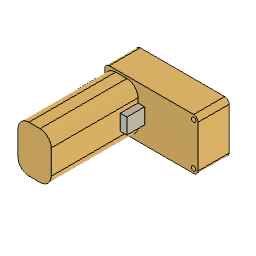
PeristalticPump_Gears (Autodesk Fusion 360 archive; units mm, degrees)
design "DC Motor from Hanka Dubovská"
part number: 2026-01-29-20-00-23-988
Autodesk Fusion 360 part; units mm, degrees
(part 1 of 2)
sketch "Sketch1" plane through (0, 0, 0) normal (0, 0, 1) x (1, 0, 0)
  line L0 (0, 0) -> (42, 0)
  line L1 (42, 0) -> (42, 14)
  line L2 (42, 14) -> (0, 14)
  line L3 (0, 14) -> (0, 0)
  line L4 (0, 0) -> (20, 0)
  dimension "d1" = 42
  dimension "d2" = 14
  constraint horizontal L0
  constraint vertical L1
  constraint horizontal L2
  constraint vertical L3
  constraint coincident L0.start L3.end
  constraint horizontal L4
  measures "d1" distance of L1.end L2.end
  measures "d2" distance of L0.end L1.end
extrude "Extrude1" add sketch "Sketch1" along normal blind 23
extrude "Extrude2" add sketch "Sketch1" along normal blind 22
sketch "Sketch3" plane through (0, 0, 0) normal (0, 1, 0) x (1, 0, 0)
  line L0 (15, -1) -> (0, -1)
  line L1 (0, -1) -> (0, -22)
  line L2 (0, -22) -> (15, -22)
  line L3 (15, -22) -> (15, -1)
  dimension "d17" = 15
  constraint horizontal L0
  constraint vertical L1
  constraint horizontal L2
  constraint vertical L3
  measures "d17" distance of L1.end L2.end
extrude "Extrude4" add sketch "Sketch3" against normal blind 39
fillet "Fillet2" radius 5 4 edges at (0, -19.5, 22) (15, -19.5, 22) (0, -19.5, 1) (15, -19.5, 1)
fillet "Fillet3" radius 2 4 edges at (0, 7, 0) (42, 7, 0) (42, 7, 23) (0, 7, 23)
sketch "Sketch4" plane through (0, 0, 0) normal (-1, 0, 0) x (0, -1, 0)
  line L0 (0, 21) -> (-14, 21)
  line L1 (-14, 21) -> (-14, 2)
  line L2 (-14, 2) -> (0, 2)
  line L3 (0, 2) -> (0, 6)
  line L4 (0, 6) -> (39, 6)
  line L5 (39, 6) -> (39, 17)
  line L6 (39, 17) -> (0, 17)
  line L7 (0, 17) -> (0, 21)
  line L8 (0, 15) -> (8, 15)
  line L9 (8, 15) -> (8, 8)
  line L10 (8, 8) -> (0, 8)
  line L11 (0, 8) -> (0, 15)
  dimension "d20" = 8
  dimension "d21" = 7
  constraint horizontal L8
  constraint vertical L9
  constraint horizontal L10
  constraint vertical L11
  measures "d20" distance of L8.start L8.end
  measures "d21" distance of L8.start L10.end
extrude "Extrude5" add sketch "Sketch4" along normal blind 4 contours L8 L9 L10 L11
sketch "Sketch5" plane through (0, 14, 0) normal (0, 1, 0) x (-1, 0, 0)
  arc A0 (0, 21) -> (-2, 23) centre (-2, 21) ccw
  line L0 (-2, 23) -> (-40, 23)
  arc A1 (-40, 23) -> (-42, 21) centre (-40, 21) ccw
  line L1 (-42, 21) -> (-42, 2)
  arc A2 (-42, 2) -> (-40, 0) centre (-40, 2) ccw
  line L2 (-40, 0) -> (-2, 0)
  arc A3 (-2, 0) -> (0, 2) centre (-2, 2) ccw
  line L3 (0, 2) -> (0, 21)
  line L4 (-30.8362, 13.6553) -> (-29.8362, 13.6553)
  line L5 (-28.8362, 12.6553) -> (-28.8362, 9.6553)
  line L6 (-29.8362, 8.6553) -> (-30.8362, 8.6553)
  line L7 (-31.8362, 9.6553) -> (-31.8362, 12.6553)
  circle A4 centre (-21, 11.5403) radius 1.5
  arc A5 (-28.8362, 12.6553) -> (-29.8362, 13.6553) centre (-29.8362, 12.6553) ccw
  arc A6 (-30.8362, 13.6553) -> (-31.8362, 12.6553) centre (-30.8362, 12.6553) ccw
  arc A7 (-31.8362, 9.6553) -> (-30.8362, 8.6553) centre (-30.8362, 9.6553) ccw
  arc A8 (-29.8362, 8.6553) -> (-28.8362, 9.6553) centre (-29.8362, 9.6553) ccw
  point P0 (-28.8362, 13.6553)
  point P1 (-28.8362, 8.6553)
  point P2 (-31.8362, 8.6553)
  dimension "d24" = 3
  dimension "d25" = 5
  dimension "d26" = 3
  dimension "d37" = 1
  constraint horizontal L4
  constraint vertical L5
  constraint horizontal L6
  constraint vertical L7
  constraint coincident P0 L4
  constraint coincident P0 L5
  constraint tangent L4 A5
  constraint tangent L5 A5
  constraint tangent L4 A6
  constraint tangent L7 A6
  constraint equal A5 A6
  constraint coincident P2 L6
  constraint coincident P2 L7
  constraint tangent L6 A7
  constraint tangent L7 A7
  constraint equal A5 A7
  constraint coincident P1 L5
  constraint coincident P1 L6
  constraint tangent L5 A8
  constraint tangent L6 A8
  constraint equal A5 A8
  measures "d24" diameter of A4
  measures "d25" distance of P0 P1
  measures "d26" distance of P1 P2
  measures "d37" radius of A5
extrude "Extrude6" add sketch "Sketch5" along normal blind 8 contours L4 L5 L6 L7 A5 A6 A7 A8
sketch "Sketch6" plane through (0, 14, 0) normal (0, 1, 0) x (-1, 0, 0)
  circle A0 centre (-21, 11.5) radius 1.5
  dimension "d29" = 3
  measures "d29" diameter of A0
extrude "Extrude7" add sketch "Sketch6" along normal blind 1
sketch "Sketch7" plane through (15, 0, 0) normal (1, 0, 0) x (0, 1, 0)
  line L0 (-39, 6) -> (0, 6)
  line L1 (0, 6) -> (0, 17)
  line L2 (0, 17) -> (-39, 17)
  line L3 (-39, 17) -> (-39, 6)
  line L4 (0, 15) -> (-8, 15)
  line L5 (-8, 15) -> (-8, 8)
  line L6 (-8, 8) -> (0, 8)
  line L7 (0, 8) -> (0, 15)
  constraint horizontal L4
  constraint vertical L5
  constraint horizontal L6
  constraint vertical L7
  constraint coincident L1 L4.start
extrude "Extrude8" add sketch "Sketch7" along normal blind 3 contours L1 L4 L5 L6 L7
sketch "Sketch8" plane through (0, 14, 0) normal (0, 1, 0) x (-1, 0, 0)
  circle A0 centre (-21, 11.5) radius 1.5
  line L0 (-31.8362, 9.6553) -> (-31.8362, 12.6553)
  line L1 (-30.8362, 13.6553) -> (-29.8362, 13.6553)
  line L2 (-28.8362, 12.6553) -> (-28.8362, 9.6553)
  line L3 (-29.8362, 8.6553) -> (-30.8362, 8.6553)
  arc A1 (0, 21) -> (-2, 23) centre (-2, 21) ccw
  line L4 (-2, 23) -> (-40, 23)
  arc A2 (-40, 23) -> (-42, 21) centre (-40, 21) ccw
  line L5 (-42, 21) -> (-42, 2)
  arc A3 (-42, 2) -> (-40, 0) centre (-40, 2) ccw
  line L6 (-40, 0) -> (-2, 0)
  arc A4 (-2, 0) -> (0, 2) centre (-2, 2) ccw
  line L7 (0, 2) -> (0, 21)
  circle A5 centre (-40, 2) radius 1
  circle A6 centre (-40, 21) radius 1
  arc A7 (-30.8362, 13.6553) -> (-31.8362, 12.6553) centre (-30.8362, 12.6553) ccw
  arc A8 (-28.8362, 12.6553) -> (-29.8362, 13.6553) centre (-29.8362, 12.6553) ccw
  arc A9 (-29.8362, 8.6553) -> (-28.8362, 9.6553) centre (-29.8362, 9.6553) ccw
  arc A10 (-31.8362, 9.6553) -> (-30.8362, 8.6553) centre (-30.8362, 9.6553) ccw
  constraint concentric A3 A5
  constraint concentric A2 A6
hole "Hole1" at (40, 14, 2) at (40, 14, 21) direction (0, -1, 0) diameter 2 depth 14 tip angle 118

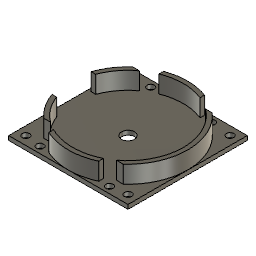
design "GearHolder"
part number: 2026-05-20-10-56-44-048
Autodesk Fusion 360 part; units mm, degrees
sketch "Sketch1" plane through (0, 0, 0) normal (0, 0, 1) x (1, 0, 0)
  line L0 (0, 55) -> (0, 0)
  circle A0 centre (51, 51) radius 1.65
  circle A1 centre (4, 51) radius 1.65
  line L1 (25, 0) -> (30, 0)
  line L2 (0, 0) -> (55, 0)
  line L3 (55, 55) -> (0, 55)
  circle A2 centre (4, 4) radius 1.65
  circle A3 centre (51, 4) radius 1.65
  line L4 (55, 0) -> (55, 55)
  line L5 (45, 55) -> (9.9854, 55)
  line L6 (45, 55) -> (38, 55)
  circle A4 centre (11.5, 3) radius 1.65
  line L7 (16.9854, 55) -> (9.9854, 55)
  circle A5 centre (43.5, 3) radius 1.65
  line L8 (8, 0) -> (47, 0)
  circle A6 centre (13.4854, 52) radius 1.65
  circle A7 centre (41.5, 52) radius 1.65
  circle A8 centre (27.5, 27.5) radius 3
  point P0 (45, 45)
  dimension "d30" = 3.3
  dimension "d31" = 4
  dimension "d32" = 4
  dimension "d33" = 3.3
  dimension "d34" = 4
  dimension "d35" = 4
  dimension "d36" = 3.3
  dimension "d37" = 4
  dimension "d38" = 4
  dimension "d39" = 3.3
  dimension "d40" = 4
  dimension "d41" = 4
  dimension "d55" = 3.3
  dimension "d56" = 3.3
  dimension "d57" = 3
  dimension "d59" = 3
  dimension "d60" = 3.3
  dimension "d61" = 3.3
  dimension "d62" = 3
  dimension "d65" = 3
  dimension "d69" = 6
  dimension "d70" = 55
  dimension "d71" = 27.5
  dimension "d72" = 55
  dimension "d73" = 27.5
  constraint horizontal L2
  constraint vertical L4
  constraint horizontal L3
  constraint vertical L0
  constraint horizontal L1
  constraint coincident L1.start L2
  constraint coincident L5.start L6.start
  constraint coincident L5.end L7.end
  measures "d30" diameter of A2
  measures "d31" distance of A2.centre L2
  measures "d32" distance of A2.centre L0
  measures "d33" diameter of A3
  measures "d34" distance of A3.centre L2
  measures "d35" distance of A3.centre L4
  measures "d36" diameter of A1
  measures "d37" distance of A1.centre L3
  measures "d38" distance of A1.centre L0
  measures "d39" diameter of A0
  measures "d40" distance of A0.centre L3
  measures "d41" distance of A0.centre L4
  measures "d55" diameter of A7
  measures "d56" diameter of A6
  measures "d57" distance of A7.centre L5
  measures "d59" distance of A6.centre L5
  measures "d60" diameter of A5
  measures "d61" diameter of A4
  measures "d62" distance of A5.centre L8
  measures "d65" distance of A4.centre L8
  measures "d69" diameter of A8
  measures "d70" distance of L0.start L0.end
  measures "d71" distance of L3 A8.centre
  measures "d72" distance of L0.start L3.start
  measures "d73" distance of L4 A8.centre
extrude "Extrude1" add sketch "Sketch1" along normal blind 2
sketch "Sketch2" plane through (0, 0, 2) normal (0, 0, 1) x (-1, 0, 0)
  line L0 (0, 0) -> (-55, 0)
  line L1 (-55, 0) -> (-55, -55)
  line L2 (-55, -55) -> (0, -55)
  line L3 (0, -55) -> (0, 0)
  circle A0 centre (-51, -51) radius 1.65
  circle A1 centre (-4, -51) radius 1.65
  circle A2 centre (-51, -4) radius 1.65
  circle A3 centre (-13.4854, -52) radius 1.65
  circle A4 centre (-43.5, -3) radius 1.65
  circle A5 centre (-4, -4) radius 1.65
  circle A6 centre (-41.5, -52) radius 1.65
  circle A7 centre (-11.5, -3) radius 1.65
  circle A8 centre (-27.5, -27.5) radius 3
  circle A9 centre (-27.5, -27.5) radius 27.5
  circle A10 centre (-27.5, -27.5) radius 25.5
  line L4 (-18, -48) -> (-8.9708, -48)
  line L5 (-8.9708, -48) -> (-8.9708, -56)
  line L6 (-8.9708, -56) -> (-18, -56)
  line L7 (-18, -56) -> (-18, -48)
  line L8 (-18, -48) -> (-8.9708, -56) construction
  line L9 (-8.9708, -48) -> (-18, -56) construction
  line L10 (-37, -48) -> (-46, -48)
  line L11 (-46, -48) -> (-46, -56)
  line L12 (-46, -56) -> (-37, -56)
  line L13 (-37, -56) -> (-37, -48)
  line L14 (-37, -48) -> (-46, -56) construction
  line L15 (-46, -48) -> (-37, -56) construction
  line L16 (-39, -7) -> (-48, -7)
  line L17 (-48, -7) -> (-48, 1)
  line L18 (-48, 1) -> (-39, 1)
  line L19 (-39, 1) -> (-39, -7)
  line L20 (-39, -7) -> (-48, 1) construction
  line L21 (-48, -7) -> (-39, 1) construction
  line L22 (-16, -7) -> (-7, -7)
  line L23 (-7, -7) -> (-7, 1)
  line L24 (-7, 1) -> (-16, 1)
  line L25 (-16, 1) -> (-16, -7)
  line L26 (-16, -7) -> (-7, 1) construction
  line L27 (-7, -7) -> (-16, 1) construction
  line L28 (0, -36.5) -> (-10, -36.5)
  line L29 (-10, -36.5) -> (-10, -18.5)
  line L30 (-10, -18.5) -> (0, -18.5)
  line L31 (0, -18.5) -> (0, -36.5)
  point P0 (-13.4854, -52)
  point P1 (-41.5, -52)
  point P2 (-43.5, -3)
  point P3 (-11.5, -3)
  dimension "d74" = 2
  dimension "d75" = 51
  dimension "d78" = 18
  dimension "d79" = 18.5
  constraint concentric A8 A9
  constraint concentric A8 A10
  constraint horizontal L4
  constraint perpendicular L4 L5
  constraint parallel L4 L6
  constraint parallel L5 L7
  constraint coincident L8 P0
  constraint coincident L9 P0
  constraint coincident P0 A3.centre
  constraint horizontal L10
  constraint perpendicular L10 L11
  constraint parallel L10 L12
  constraint parallel L11 L13
  constraint coincident L14 P1
  constraint coincident L15 P1
  constraint coincident P1 A6.centre
  constraint horizontal L16
  constraint perpendicular L16 L17
  constraint parallel L16 L18
  constraint parallel L17 L19
  constraint coincident L20 P2
  constraint coincident L21 P2
  constraint coincident P2 A4.centre
  constraint horizontal L22
  constraint perpendicular L22 L23
  constraint parallel L22 L24
  constraint parallel L23 L25
  constraint coincident L26 P3
  constraint coincident L27 P3
  constraint coincident P3 A7.centre
  constraint horizontal L28
  constraint vertical L29
  constraint horizontal L30
  constraint vertical L31
  constraint coincident L3 L28.start
  measures "d74" distance of A9 A10
  measures "d75" diameter of A10
  measures "d78" distance of L28.end L29.end
  measures "d79" distance of L2.end L28.start
extrude "Extrude2" add sketch "Sketch2" along normal blind 8 contours A9 A10 L22 L30 | A9 A10 L19 L25 | A9 A10 L4 L28 | A9 A10 L10 L16 | A9 A10 L7 L13

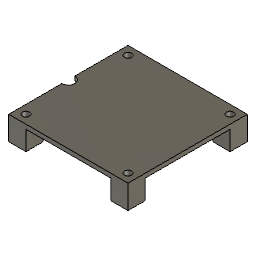
design "GearHolderP2"
part number: 2026-05-20-11-23-21-013
Autodesk Fusion 360 part; units mm, degrees
sketch "Sketch1" plane through (0, 0, 0) normal (0, 0, 1) x (1, 0, 0)
  circle A0 centre (51, 4) radius 1.65
  line L0 (16.9854, 55) -> (9.9854, 55)
  line L1 (0, 55) -> (0, 0)
  circle A1 centre (4, 4) radius 1.65
  line L2 (25, 0) -> (30, 0)
  line L3 (8, 0) -> (47, 0)
  line L4 (55, 0) -> (55, 55)
  line L5 (0, 0) -> (55, 0)
  line L6 (45, 55) -> (38, 55)
  line L7 (55, 55) -> (0, 55)
  circle A2 centre (51, 51) radius 1.65
  circle A3 centre (4, 51) radius 1.65
  line L8 (45, 55) -> (9.9854, 55)
  line L9 (0, 55) -> (8, 55)
  line L10 (8, 55) -> (8, 47)
  line L11 (8, 47) -> (0, 47)
  line L12 (0, 47) -> (0, 55)
  line L13 (0, 55) -> (8, 47) construction
  line L14 (8, 55) -> (0, 47) construction
  line L15 (55, 55) -> (47, 55)
  line L16 (47, 55) -> (47, 47)
  line L17 (47, 47) -> (55, 47)
  line L18 (55, 47) -> (55, 55)
  line L19 (55, 55) -> (47, 47) construction
  line L20 (47, 55) -> (55, 47) construction
  line L21 (55, 0) -> (47, 0)
  line L22 (47, 0) -> (47, 8)
  line L23 (47, 8) -> (55, 8)
  line L24 (55, 8) -> (55, 0)
  line L25 (55, 0) -> (47, 8) construction
  line L26 (47, 0) -> (55, 8) construction
  line L27 (0, 0) -> (8, 0)
  line L28 (8, 0) -> (8, 8)
  line L29 (8, 8) -> (0, 8)
  line L30 (0, 8) -> (0, 0)
  line L31 (0, 0) -> (8, 8) construction
  line L32 (8, 0) -> (0, 8) construction
  circle A4 centre (0, 27.5) radius 3
  point P0 (45, 45)
  point P1 (4, 51)
  point P2 (51, 51)
  point P3 (51, 4)
  point P4 (4, 4)
  dimension "d1" = 3.3
  dimension "d2" = 4
  dimension "d3" = 4
  dimension "d4" = 3.3
  dimension "d5" = 4
  dimension "d6" = 4
  dimension "d7" = 3.3
  dimension "d8" = 4
  dimension "d9" = 4
  dimension "d10" = 3.3
  dimension "d11" = 4
  dimension "d12" = 4
  dimension "d22" = 55
  dimension "d24" = 55
  dimension "d31" = 6
  dimension "d32" = 27.5
  constraint horizontal L5
  constraint vertical L4
  constraint horizontal L7
  constraint vertical L1
  constraint horizontal L2
  constraint coincident L2.start L5
  constraint coincident L6.start L8.start
  constraint coincident L0.end L8.end
  constraint horizontal L9
  constraint perpendicular L9 L10
  constraint parallel L9 L11
  constraint parallel L10 L12
  constraint coincident L13 P1
  constraint coincident L14 P1
  constraint coincident P1 A3.centre
  constraint horizontal L15
  constraint perpendicular L15 L16
  constraint parallel L15 L17
  constraint parallel L16 L18
  constraint coincident L19 P2
  constraint coincident L20 P2
  constraint coincident P2 A2.centre
  constraint horizontal L21
  constraint perpendicular L21 L22
  constraint parallel L21 L23
  constraint parallel L22 L24
  constraint coincident L25 P3
  constraint coincident L26 P3
  constraint coincident A0.centre P3
  constraint horizontal L27
  constraint perpendicular L27 L28
  constraint parallel L27 L29
  constraint parallel L28 L30
  constraint coincident L31 P4
  constraint coincident L32 P4
  constraint coincident L1.end L5.start
  constraint coincident P4 A1.centre
  constraint coincident L1 A4.centre
  measures "d1" diameter of A1
  measures "d2" distance of P4 L5
  measures "d3" distance of P4 L1
  measures "d4" diameter of A0
  measures "d5" distance of A0.centre L5
  measures "d6" distance of A0.centre L4
  measures "d7" diameter of A3
  measures "d8" distance of P1 L7
  measures "d9" distance of P1 L1
  measures "d10" diameter of A2
  measures "d11" distance of P2 L7
  measures "d12" distance of P2 L4
  measures "d22" distance of L1.start L1.end
  measures "d24" distance of L1.start L4.end
  measures "d31" diameter of A4
  measures "d32" distance of L1.start A4.centre
extrude "Extrude1" add sketch "Sketch1" along normal blind 9 contours L1 L7 L9 L10 L11 L12 | L4 L7 L15 L16 L17 L18 | L4 L5 L21 L22 L23 L24 | L1 L5 L27 L28 L29 L30 makes body 1 at (50.1048, 49.614, 6) makes body 2 at (51.8952, 2.614, 3) makes body 3 at (5.6173, 50.6731, 6) makes body 4 at (5.6479, 3.9178, 6)
extrude "Extrude2" add sketch "Sketch1" along normal blind 2 from surface at 9 contours L0 L1 L2 L3 L4 L5 L6 L7 L8 L10 L11 L16 L17 L22 L23 L28 L29 A4 | L1 L7 L9 L10 L11 L12 | L4 L7 L15 L16 L17 L18 | L4 L5 L21 L22 L23 L24 | L1 L5 L27 L28 L29 L30 bodies 1 2 3 4

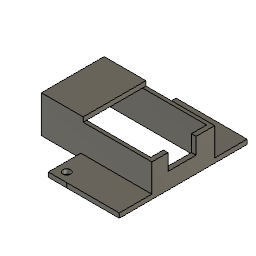
design "GearHolderP3"
part number: 2026-05-20-11-42-52-176
Autodesk Fusion 360 part; units mm, degrees
sketch "Sketch1" plane through (0, 0, 0) normal (0, 0, 1) x (1, 0, 0)
  line L0 (0, 55) -> (-8, 47) construction
  circle A0 centre (-4.0079, 4.0002) radius 1.65
  line L1 (-0.0158, 8.0004) -> (-8, 8.0004)
  line L2 (-8, 0) -> (-0.0158, 8.0004) construction
  line L3 (-0.0158, 0) -> (-8, 8.0004) construction
  line L4 (-0.0158, 0) -> (-0.0158, 8.0004)
  line L5 (0, 55) -> (0, 47)
  line L6 (-8, 0) -> (-0.0158, 0)
  line L7 (-8, 8.0004) -> (-8, 0)
  line L8 (-8, 47) -> (-8, 55)
  circle A1 centre (-4, 51) radius 1.65
  line L9 (-8, 55) -> (0, 47) construction
  line L10 (-8, 55) -> (0, 55)
  line L11 (0, 47) -> (-8, 47)
  line L12 (20.5318, 39.5004) -> (20.5318, 15.5004)
  line L13 (20.5318, 39.5004) -> (-23, 39.5004)
  line L14 (-22.9682, 39.5004) -> (-22.9682, 15.5004)
  line L15 (-22.9682, 15.5004) -> (20.5318, 15.5004)
  line L16 (-24.9682, 41.0004) -> (22.5318, 41.0004)
  line L17 (22.5318, 41.0004) -> (22.5318, 14.0004)
  line L18 (22.5318, 14.0004) -> (-24.9682, 14.0004)
  line L19 (-24.9682, 14.0004) -> (-24.9682, 41.0004)
  line L20 (-6.9682, 41.0004) -> (-6.9682, 14.0004)
  line L21 (-8, 47) -> (-8, 41)
  line L22 (-8, 8.0004) -> (-8, 14.0004)
  line L23 (22.5318, 41.0004) -> (22.5318, 54.9634)
  line L24 (22.5318, 54.9634) -> (0, 55)
  line L25 (22.5318, 14.0004) -> (22.5318, -0.0052)
  line L26 (22.5318, -0.0052) -> (-0.0158, 0)
  line L27 (20.5318, 33) -> (22.5318, 33)
  line L28 (22.5318, 33) -> (22.5318, 21)
  line L29 (22.5318, 21) -> (20.5318, 21)
  line L30 (20.5318, 21) -> (20.5318, 33)
  point P0 (-8, 0)
  point P1 (-4, 51)
  point P2 (-4.0079, 4.0002)
  point P3 (9.9854, 55)
  point P4 (9.9854, 55)
  point P5 (-7.9947, 0.536)
  point P6 (-0.0158, 0)
  dimension "d1" = 3.3
  dimension "d3" = 3.3
  dimension "d6" = 24
  dimension "d8" = 1.5
  dimension "d9" = 2
  dimension "d10" = 1.5
  dimension "d11" = 2
  dimension "d12" = 16
  dimension "d14" = 8
  dimension "d15" = 8
  dimension "d18" = 6
  dimension "d19" = 6
  dimension "d20" = 8.0004
  dimension "d30" = 43.5
  constraint coincident P4 P3
  constraint horizontal L10
  constraint perpendicular L5 L10
  constraint parallel L10 L11
  constraint parallel L5 L8
  constraint coincident P1 L9
  constraint coincident P1 L0
  constraint coincident P1 A1.centre
  constraint horizontal L6
  constraint perpendicular L4 L6
  constraint parallel L1 L6
  constraint parallel L4 L7
  constraint coincident P2 L2
  constraint coincident P2 L3
  constraint coincident P0 L2.start
  constraint coincident P2 A0.centre
  constraint perpendicular L12 L13
  constraint coincident L13 L14.start
  constraint perpendicular L13 L14
  constraint horizontal L16
  constraint vertical L17
  constraint horizontal L18
  constraint vertical L19
  constraint coincident L16 L20.start
  constraint coincident L18 L20.end
  constraint perpendicular L18 L20
  constraint perpendicular L16 L21
  constraint coincident L18 L22.end
  constraint perpendicular L18 L22
  constraint perpendicular L16 L23
  constraint perpendicular L18 L25
  constraint coincident P6 L3.start
  constraint horizontal L27
  constraint vertical L28
  constraint horizontal L29
  constraint vertical L30
  constraint coincident L17 L28.end
  constraint coincident L12 L27.start
  measures "d1" diameter of A0
  measures "d3" diameter of A1
  measures "d6" distance of L12.start L12.end
  measures "d8" distance of L13 L16
  measures "d9" distance of L12 L17
  measures "d10" distance of L15 L18
  measures "d11" distance of L14 L19
  measures "d12" distance of L14 L20
  measures "d14" distance of L8.end L0.start
  measures "d15" distance of L8.end L0.end
  measures "d18" distance of L0.end L21.end
  measures "d19" distance of L1.end L22.end
  measures "d20" distance of L1.end P0
  measures "d30" distance of L12 L14
extrude "Extrude1" add sketch "Sketch1" along normal blind 2 contours L1 L4 L6 L7 | L1 L4 L18 L22 L25 L26 | L5 L11 L16 L21 L23 L24 | L5 L8 L10 L11 makes body 1 at (15.0212, 50.3213, 0) makes body 2 at (15.0159, 4.6651, 0)
extrude "Extrude2" add sketch "Sketch1" along normal blind 14 contours L13 L14 L15 L16 L18 L19 L20 | L12 L15 L17 L18 L20 L29 | L12 L13 L16 L17 L20 L27 bodies 1 2
extrude "Extrude3" add sketch "Sketch1" along normal blind 2 from surface at 14 contours L13 L14 L15 L16 L18 L19 L20 | L13 L14 L15 L20 bodies 1
extrude "Extrude4" add sketch "Sketch1" along normal blind 7 contours L12 L17 L27 L28 L29 L30 bodies 1

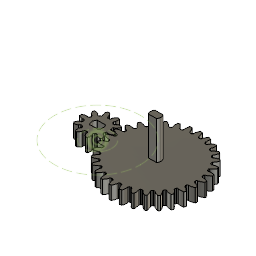
design "MotorGearsV3"
description: Spur Gear; Module: 1.5; Num Teeth: 30; Pressure Angle: 20.0; Backlash: 0.00 mm
part number: 2026-05-20-09-17-09-807
Autodesk Fusion 360 part; units mm, degrees
sketch "Base Circle" plane through (0, 0, 0) normal (0, 0, 1) x (1, 0, 0)
  circle A0 centre (0, 0) radius 5.7645
extrude "Extrude1" add sketch "Base Circle" along normal blind 7 makes body 1
sketch "Gear Tooth" plane through (0, 0, 0) normal (0, 0, 1) x (1, 0, 0)
  spline S0 degree 5 poles (6.9437, -1.2061) (6.9494, -1.2071) (6.9609, -1.2089) (6.9781, -1.211) (7.0011, -1.2127) (7.0301, -1.2132) (7.0593, -1.2127) (7.0885, -1.2115) (7.1178, -1.2099) (7.1471, -1.208) (7.1764, -1.2059) (7.2058, -1.2034) (7.2353, -1.2005) (7.2647, -1.197) (7.2943, -1.1929) (7.3238, -1.1884) (7.3534, -1.1833) (7.383, -1.178) (7.4126, -1.1723) (7.4422, -1.1663) (7.4719, -1.1599) (7.5015, -1.1533) (7.5312, -1.1463) (7.5609, -1.139) (7.5906, -1.1313) (7.6202, -1.1232) (7.6499, -1.1148) (7.6796, -1.1062) (7.7093, -1.0972) (7.7389, -1.0879) (7.7686, -1.0784) (7.7983, -1.0685) (7.8279, -1.0584) (7.8575, -1.048) (7.8872, -1.0372) (7.9168, -1.0262) (7.9464, -1.015) (7.9759, -1.0034) (8.0055, -0.9916) (8.035, -0.9795) (8.0645, -0.9671) (8.094, -0.9545) (8.1235, -0.9416) (8.1529, -0.9284) (8.1823, -0.915) (8.2117, -0.9013) (8.241, -0.8874) (8.2704, -0.8732) (8.2996, -0.8587) (8.3289, -0.844) (8.3581, -0.8291) (8.3873, -0.8139) (8.4164, -0.7985) (8.4455, -0.7828) (8.4746, -0.7669) (8.5036, -0.7508) (8.5325, -0.7344) (8.5615, -0.7177) (8.5903, -0.7009) (8.6192, -0.6838) (8.648, -0.6664) (8.6767, -0.6489) (8.7054, -0.6311) (8.734, -0.613) (8.7626, -0.5948) (8.7911, -0.5763) (8.8196, -0.5576) (8.848, -0.5387) (8.8764, -0.5195) (8.9047, -0.5001) (8.9329, -0.4805) (8.9555, -0.4647) (8.9723, -0.4527) (8.9836, -0.4446) (8.9892, -0.4406) knots 0 0 0 0 0 0 0.01428571 0.02857143 0.04285714 0.05714286 0.07142857 0.08571429 0.1 0.11428571 0.12857143 0.14285714 0.15714286 0.17142857 0.18571429 0.2 0.21428571 0.22857143 0.24285714 0.25714286 0.27142857 0.28571429 0.3 0.31428571 0.32857143 0.34285714 0.35714286 0.37142857 0.38571429 0.4 0.41428571 0.42857143 0.44285714 0.45714286 0.47142857 0.48571429 0.5 0.51428571 0.52857143 0.54285714 0.55714286 0.57142857 0.58571429 0.6 0.61428571 0.62857143 0.64285714 0.65714286 0.67142857 0.68571429 0.7 0.71428571 0.72857143 0.74285714 0.75714286 0.77142857 0.78571429 0.8 0.81428571 0.82857143 0.84285714 0.85714286 0.87142857 0.88571429 0.9 0.91428571 0.92857143 0.94285714 0.95714286 0.97142857 0.98571429 1 1 1 1 1 1
  spline S1 degree 5 poles (6.9437, 1.2061) (6.9494, 1.2071) (6.9609, 1.2089) (6.9781, 1.211) (7.0011, 1.2127) (7.0301, 1.2132) (7.0593, 1.2127) (7.0885, 1.2115) (7.1178, 1.2099) (7.1471, 1.208) (7.1764, 1.2059) (7.2058, 1.2034) (7.2353, 1.2005) (7.2647, 1.197) (7.2943, 1.1929) (7.3238, 1.1884) (7.3534, 1.1833) (7.383, 1.178) (7.4126, 1.1723) (7.4422, 1.1663) (7.4719, 1.1599) (7.5015, 1.1533) (7.5312, 1.1463) (7.5609, 1.139) (7.5906, 1.1313) (7.6202, 1.1232) (7.6499, 1.1148) (7.6796, 1.1062) (7.7093, 1.0972) (7.7389, 1.0879) (7.7686, 1.0784) (7.7983, 1.0685) (7.8279, 1.0584) (7.8575, 1.048) (7.8872, 1.0372) (7.9168, 1.0262) (7.9464, 1.015) (7.9759, 1.0034) (8.0055, 0.9916) (8.035, 0.9795) (8.0645, 0.9671) (8.094, 0.9545) (8.1235, 0.9416) (8.1529, 0.9284) (8.1823, 0.915) (8.2117, 0.9013) (8.241, 0.8874) (8.2704, 0.8732) (8.2996, 0.8587) (8.3289, 0.844) (8.3581, 0.8291) (8.3873, 0.8139) (8.4164, 0.7985) (8.4455, 0.7828) (8.4746, 0.7669) (8.5036, 0.7508) (8.5325, 0.7344) (8.5615, 0.7177) (8.5903, 0.7009) (8.6192, 0.6838) (8.648, 0.6664) (8.6767, 0.6489) (8.7054, 0.6311) (8.734, 0.613) (8.7626, 0.5948) (8.7911, 0.5763) (8.8196, 0.5576) (8.848, 0.5387) (8.8764, 0.5195) (8.9047, 0.5001) (8.9329, 0.4805) (8.9555, 0.4647) (8.9723, 0.4527) (8.9836, 0.4446) (8.9892, 0.4406) knots 0 0 0 0 0 0 0.01428571 0.02857143 0.04285714 0.05714286 0.07142857 0.08571429 0.1 0.11428571 0.12857143 0.14285714 0.15714286 0.17142857 0.18571429 0.2 0.21428571 0.22857143 0.24285714 0.25714286 0.27142857 0.28571429 0.3 0.31428571 0.32857143 0.34285714 0.35714286 0.37142857 0.38571429 0.4 0.41428571 0.42857143 0.44285714 0.45714286 0.47142857 0.48571429 0.5 0.51428571 0.52857143 0.54285714 0.55714286 0.57142857 0.58571429 0.6 0.61428571 0.62857143 0.64285714 0.65714286 0.67142857 0.68571429 0.7 0.71428571 0.72857143 0.74285714 0.75714286 0.77142857 0.78571429 0.8 0.81428571 0.82857143 0.84285714 0.85714286 0.87142857 0.88571429 0.9 0.91428571 0.92857143 0.94285714 0.95714286 0.97142857 0.98571429 1 1 1 1 1 1
  arc A0 (8.9892, -0.4406) -> (8.9892, 0.4406) centre (0, 0) ccw
  line L0 (5.6696, -0.9848) -> (6.9437, -1.2061)
  line L1 (5.6696, 0.9848) -> (6.9437, 1.2061)
  line L2 (5.6696, -0.9848) -> (5.6696, 0.9848)
  point P0 (7.0843, -1.2116)
  point P1 (7.2275, -1.2012)
  point P2 (7.3722, -1.1799)
  point P3 (7.5182, -1.1493)
  point P4 (7.6649, -1.1104)
  point P5 (7.8123, -1.0637)
  point P6 (7.9601, -1.0096)
  point P7 (8.108, -0.9483)
  point P8 (8.256, -0.8801)
  point P9 (8.4037, -0.8052)
  point P10 (8.5511, -0.7237)
  point P11 (8.6979, -0.6357)
  point P12 (8.844, -0.5413)
  point P13 (7.0843, 1.2116)
  point P14 (7.2275, 1.2012)
  point P15 (7.3722, 1.1799)
  point P16 (7.5182, 1.1493)
  point P17 (7.6649, 1.1104)
  point P18 (7.8123, 1.0637)
  point P19 (7.9601, 1.0096)
  point P20 (8.108, 0.9483)
  point P21 (8.256, 0.8801)
  point P22 (8.4037, 0.8052)
  point P23 (8.5511, 0.7237)
  point P24 (8.6979, 0.6357)
  point P25 (8.844, 0.5413)
extrude "Extrude2" add sketch "Gear Tooth" along normal blind 7 bodies 1
fillet "Fillet1" radius 0.5 2 edges at (5.6795, -0.9865, 3.5) (5.6795, 0.9865, 3.5) on bodies 1
pattern_circular "C-Pattern1" count 10 over 360 about axis through (0, 0, 0) along (0, 0, 1) of "Extrude2", "Fillet1"
sketch "Diametrial Pitch Circle" plane through (0, 0, 0) normal (0, 0, 1) x (1, 0, 0)
  circle A0 centre (0, 0) radius 7.5 construction
sketch "Base Circle (1)" plane through (0, 0, 0) normal (0, 0, 1) x (1, 0, 0)
  circle A0 centre (0, 0) radius 20.7645
extrude "Extrude3" add sketch "Base Circle (1)" along normal blind 7 separate body makes body 2
sketch "Gear Tooth (1)" plane through (0, 0, 0) normal (0, 0, 1) x (1, 0, 0)
  spline S0 degree 5 poles (21.0953, -1.4211) (21.1036, -1.4217) (21.1202, -1.4226) (21.1452, -1.4234) (21.1786, -1.4233) (21.2203, -1.4217) (21.262, -1.419) (21.3037, -1.4156) (21.3455, -1.4119) (21.3873, -1.4079) (21.4291, -1.4036) (21.4709, -1.399) (21.5127, -1.3939) (21.5545, -1.3883) (21.5963, -1.3822) (21.6381, -1.3756) (21.6799, -1.3685) (21.7217, -1.3611) (21.7635, -1.3534) (21.8052, -1.3454) (21.847, -1.3371) (21.8888, -1.3285) (21.9306, -1.3196) (21.9723, -1.3103) (22.014, -1.3008) (22.0558, -1.2909) (22.0975, -1.2807) (22.1392, -1.2702) (22.1809, -1.2594) (22.2225, -1.2484) (22.2642, -1.2371) (22.3059, -1.2255) (22.3475, -1.2137) (22.3891, -1.2016) (22.4307, -1.1893) (22.4723, -1.1767) (22.5138, -1.1638) (22.5554, -1.1507) (22.5969, -1.1374) (22.6384, -1.1238) (22.6799, -1.11) (22.7213, -1.0959) (22.7628, -1.0816) (22.8042, -1.0671) (22.8456, -1.0523) (22.887, -1.0373) (22.9283, -1.0221) (22.9696, -1.0067) (23.0109, -0.991) (23.0522, -0.9751) (23.0934, -0.959) (23.1347, -0.9427) (23.1759, -0.9262) (23.217, -0.9095) (23.2582, -0.8925) (23.2993, -0.8754) (23.3404, -0.858) (23.3814, -0.8404) (23.4225, -0.8226) (23.4635, -0.8047) (23.5044, -0.7865) (23.5454, -0.7681) (23.5863, -0.7495) (23.6272, -0.7308) (23.668, -0.7118) (23.7088, -0.6926) (23.7496, -0.6732) (23.7904, -0.6537) (23.8311, -0.6339) (23.8718, -0.614) (23.9124, -0.5939) (23.9449, -0.5776) (23.9693, -0.5653) (23.9855, -0.5571) (23.9936, -0.553) knots 0 0 0 0 0 0 0.01428571 0.02857143 0.04285714 0.05714286 0.07142857 0.08571429 0.1 0.11428571 0.12857143 0.14285714 0.15714286 0.17142857 0.18571429 0.2 0.21428571 0.22857143 0.24285714 0.25714286 0.27142857 0.28571429 0.3 0.31428571 0.32857143 0.34285714 0.35714286 0.37142857 0.38571429 0.4 0.41428571 0.42857143 0.44285714 0.45714286 0.47142857 0.48571429 0.5 0.51428571 0.52857143 0.54285714 0.55714286 0.57142857 0.58571429 0.6 0.61428571 0.62857143 0.64285714 0.65714286 0.67142857 0.68571429 0.7 0.71428571 0.72857143 0.74285714 0.75714286 0.77142857 0.78571429 0.8 0.81428571 0.82857143 0.84285714 0.85714286 0.87142857 0.88571429 0.9 0.91428571 0.92857143 0.94285714 0.95714286 0.97142857 0.98571429 1 1 1 1 1 1
  spline S1 degree 5 poles (21.0953, 1.4211) (21.1036, 1.4217) (21.1202, 1.4226) (21.1452, 1.4234) (21.1786, 1.4233) (21.2203, 1.4217) (21.262, 1.419) (21.3037, 1.4156) (21.3455, 1.4119) (21.3873, 1.4079) (21.4291, 1.4036) (21.4709, 1.399) (21.5127, 1.3939) (21.5545, 1.3883) (21.5963, 1.3822) (21.6381, 1.3756) (21.6799, 1.3685) (21.7217, 1.3611) (21.7635, 1.3534) (21.8052, 1.3454) (21.847, 1.3371) (21.8888, 1.3285) (21.9306, 1.3196) (21.9723, 1.3103) (22.014, 1.3008) (22.0558, 1.2909) (22.0975, 1.2807) (22.1392, 1.2702) (22.1809, 1.2594) (22.2225, 1.2484) (22.2642, 1.2371) (22.3059, 1.2255) (22.3475, 1.2137) (22.3891, 1.2016) (22.4307, 1.1893) (22.4723, 1.1767) (22.5138, 1.1638) (22.5554, 1.1507) (22.5969, 1.1374) (22.6384, 1.1238) (22.6799, 1.11) (22.7213, 1.0959) (22.7628, 1.0816) (22.8042, 1.0671) (22.8456, 1.0523) (22.887, 1.0373) (22.9283, 1.0221) (22.9696, 1.0067) (23.0109, 0.991) (23.0522, 0.9751) (23.0934, 0.959) (23.1347, 0.9427) (23.1759, 0.9262) (23.217, 0.9095) (23.2582, 0.8925) (23.2993, 0.8754) (23.3404, 0.858) (23.3814, 0.8404) (23.4225, 0.8226) (23.4635, 0.8047) (23.5044, 0.7865) (23.5454, 0.7681) (23.5863, 0.7495) (23.6272, 0.7308) (23.668, 0.7118) (23.7088, 0.6926) (23.7496, 0.6732) (23.7904, 0.6537) (23.8311, 0.6339) (23.8718, 0.614) (23.9124, 0.5939) (23.9449, 0.5776) (23.9693, 0.5653) (23.9855, 0.5571) (23.9936, 0.553) knots 0 0 0 0 0 0 0.01428571 0.02857143 0.04285714 0.05714286 0.07142857 0.08571429 0.1 0.11428571 0.12857143 0.14285714 0.15714286 0.17142857 0.18571429 0.2 0.21428571 0.22857143 0.24285714 0.25714286 0.27142857 0.28571429 0.3 0.31428571 0.32857143 0.34285714 0.35714286 0.37142857 0.38571429 0.4 0.41428571 0.42857143 0.44285714 0.45714286 0.47142857 0.48571429 0.5 0.51428571 0.52857143 0.54285714 0.55714286 0.57142857 0.58571429 0.6 0.61428571 0.62857143 0.64285714 0.65714286 0.67142857 0.68571429 0.7 0.71428571 0.72857143 0.74285714 0.75714286 0.77142857 0.78571429 0.8 0.81428571 0.82857143 0.84285714 0.85714286 0.87142857 0.88571429 0.9 0.91428571 0.92857143 0.94285714 0.95714286 0.97142857 0.98571429 1 1 1 1 1 1
  arc A0 (23.9936, -0.553) -> (23.9936, 0.553) centre (0, 0) ccw
  line L0 (20.7076, -1.395) -> (21.0953, -1.4211)
  line L1 (20.7076, 1.395) -> (21.0953, 1.4211)
  line L2 (20.7076, -1.395) -> (20.7076, 1.395)
  point P0 (21.3001, -1.4159)
  point P1 (21.506, -1.3946)
  point P2 (21.7126, -1.3627)
  point P3 (21.9195, -1.3219)
  point P4 (22.1268, -1.2732)
  point P5 (22.3343, -1.2174)
  point P6 (22.542, -1.1549)
  point P7 (22.7497, -1.0861)
  point P8 (22.9574, -1.0112)
  point P9 (23.1651, -0.9305)
  point P10 (23.3726, -0.8442)
  point P11 (23.5799, -0.7524)
  point P12 (23.7869, -0.6553)
  point P13 (21.3001, 1.4159)
  point P14 (21.506, 1.3946)
  point P15 (21.7126, 1.3627)
  point P16 (21.9195, 1.3219)
  point P17 (22.1268, 1.2732)
  point P18 (22.3343, 1.2174)
  point P19 (22.542, 1.1549)
  point P20 (22.7497, 1.0861)
  point P21 (22.9574, 1.0112)
  point P22 (23.1651, 0.9305)
  point P23 (23.3726, 0.8442)
  point P24 (23.5799, 0.7524)
  point P25 (23.7869, 0.6553)
extrude "Extrude4" add sketch "Gear Tooth (1)" along normal blind 7 bodies 2
fillet "Fillet2" radius 0.5 2 edges at (20.7175, -1.3957, 3.5) (20.7175, 1.3957, 3.5) on bodies 2
pattern_circular "C-Pattern2" count 30 over 360 about axis through (0, 0, -0.0003) along (0, 0, 1) of "Extrude4", "Fillet2"
sketch "Diametrial Pitch Circle (1)" plane through (0, 0, 0) normal (0, 0, 1) x (1, 0, 0)
  circle A0 centre (0, 0) radius 22.5 construction
move_body "Move1" bodies 2 to x (0.994522, 0.104528, 0) y (-0.104528, 0.994522, 0) z (0, 0, 1) at (30.6, 0, 0)
sketch "Sketch7" plane through (0, 0, 7) normal (0, 0, 1) x (-1, 0, 0)
  arc A0 (-5.3609, 2.1191) -> (-5.5826, 1.4367) centre (0, 0) ccw
  arc A1 (-6.1524, 1.0687) -> (-5.5826, 1.4367) centre (-6.0668, 1.5613) ccw
  line L0 (-6.1524, 1.0687) -> (-6.9437, 1.2061)
  spline S0 degree 5 poles (-6.9437, 1.2061) (-6.9494, 1.2071) (-6.9609, 1.2089) (-6.9781, 1.211) (-7.0011, 1.2127) (-7.0301, 1.2132) (-7.0593, 1.2127) (-7.0885, 1.2115) (-7.1178, 1.2099) (-7.1471, 1.208) (-7.1764, 1.2059) (-7.2058, 1.2034) (-7.2353, 1.2005) (-7.2647, 1.197) (-7.2943, 1.1929) (-7.3238, 1.1884) (-7.3534, 1.1833) (-7.383, 1.178) (-7.4126, 1.1723) (-7.4422, 1.1663) (-7.4719, 1.1599) (-7.5015, 1.1533) (-7.5312, 1.1463) (-7.5609, 1.139) (-7.5906, 1.1313) (-7.6202, 1.1232) (-7.6499, 1.1148) (-7.6796, 1.1062) (-7.7093, 1.0972) (-7.7389, 1.0879) (-7.7686, 1.0784) (-7.7983, 1.0685) (-7.8279, 1.0584) (-7.8575, 1.048) (-7.8872, 1.0372) (-7.9168, 1.0262) (-7.9464, 1.015) (-7.9759, 1.0034) (-8.0055, 0.9916) (-8.035, 0.9795) (-8.0645, 0.9671) (-8.094, 0.9545) (-8.1235, 0.9416) (-8.1529, 0.9284) (-8.1823, 0.915) (-8.2117, 0.9013) (-8.241, 0.8874) (-8.2704, 0.8732) (-8.2996, 0.8587) (-8.3289, 0.844) (-8.3581, 0.8291) (-8.3873, 0.8139) (-8.4164, 0.7985) (-8.4455, 0.7828) (-8.4746, 0.7669) (-8.5036, 0.7508) (-8.5325, 0.7344) (-8.5615, 0.7177) (-8.5903, 0.7009) (-8.6192, 0.6838) (-8.648, 0.6664) (-8.6767, 0.6489) (-8.7054, 0.6311) (-8.734, 0.613) (-8.7626, 0.5948) (-8.7911, 0.5763) (-8.8196, 0.5576) (-8.848, 0.5387) (-8.8764, 0.5195) (-8.9047, 0.5001) (-8.9329, 0.4805) (-8.9555, 0.4647) (-8.9723, 0.4527) (-8.9836, 0.4446) (-8.9892, 0.4406) knots 0 0 0 0 0 0 0.01428571 0.02857143 0.04285714 0.05714286 0.07142857 0.08571429 0.1 0.11428571 0.12857143 0.14285714 0.15714286 0.17142857 0.18571429 0.2 0.21428571 0.22857143 0.24285714 0.25714286 0.27142857 0.28571429 0.3 0.31428571 0.32857143 0.34285714 0.35714286 0.37142857 0.38571429 0.4 0.41428571 0.42857143 0.44285714 0.45714286 0.47142857 0.48571429 0.5 0.51428571 0.52857143 0.54285714 0.55714286 0.57142857 0.58571429 0.6 0.61428571 0.62857143 0.64285714 0.65714286 0.67142857 0.68571429 0.7 0.71428571 0.72857143 0.74285714 0.75714286 0.77142857 0.78571429 0.8 0.81428571 0.82857143 0.84285714 0.85714286 0.87142857 0.88571429 0.9 0.91428571 0.92857143 0.94285714 0.95714286 0.97142857 0.98571429 1 1 1 1 1 1
  arc A2 (-8.9892, 0.4406) -> (-8.9892, -0.4406) centre (0, 0) ccw
  spline S1 degree 5 poles (-8.9892, -0.4406) (-8.9836, -0.4446) (-8.9723, -0.4527) (-8.9555, -0.4647) (-8.9329, -0.4805) (-8.9047, -0.5001) (-8.8764, -0.5195) (-8.848, -0.5387) (-8.8196, -0.5576) (-8.7911, -0.5763) (-8.7626, -0.5948) (-8.734, -0.613) (-8.7054, -0.6311) (-8.6767, -0.6489) (-8.648, -0.6664) (-8.6192, -0.6838) (-8.5903, -0.7009) (-8.5615, -0.7177) (-8.5325, -0.7344) (-8.5036, -0.7508) (-8.4746, -0.7669) (-8.4455, -0.7828) (-8.4164, -0.7985) (-8.3873, -0.8139) (-8.3581, -0.8291) (-8.3289, -0.844) (-8.2996, -0.8587) (-8.2704, -0.8732) (-8.241, -0.8874) (-8.2117, -0.9013) (-8.1823, -0.915) (-8.1529, -0.9284) (-8.1235, -0.9416) (-8.094, -0.9545) (-8.0645, -0.9671) (-8.035, -0.9795) (-8.0055, -0.9916) (-7.9759, -1.0034) (-7.9464, -1.015) (-7.9168, -1.0262) (-7.8872, -1.0372) (-7.8575, -1.048) (-7.8279, -1.0584) (-7.7983, -1.0685) (-7.7686, -1.0784) (-7.7389, -1.0879) (-7.7093, -1.0972) (-7.6796, -1.1062) (-7.6499, -1.1148) (-7.6202, -1.1232) (-7.5906, -1.1313) (-7.5609, -1.139) (-7.5312, -1.1463) (-7.5015, -1.1533) (-7.4719, -1.1599) (-7.4422, -1.1663) (-7.4126, -1.1723) (-7.383, -1.178) (-7.3534, -1.1833) (-7.3238, -1.1884) (-7.2943, -1.1929) (-7.2647, -1.197) (-7.2353, -1.2005) (-7.2058, -1.2034) (-7.1764, -1.2059) (-7.1471, -1.208) (-7.1178, -1.2099) (-7.0885, -1.2115) (-7.0593, -1.2127) (-7.0301, -1.2132) (-7.0011, -1.2127) (-6.9781, -1.211) (-6.9609, -1.2089) (-6.9494, -1.2071) (-6.9437, -1.2061) knots -1 -1 -1 -1 -1 -1 -0.98571429 -0.97142857 -0.95714286 -0.94285714 -0.92857143 -0.91428571 -0.9 -0.88571429 -0.87142857 -0.85714286 -0.84285714 -0.82857143 -0.81428571 -0.8 -0.78571429 -0.77142857 -0.75714286 -0.74285714 -0.72857143 -0.71428571 -0.7 -0.68571429 -0.67142857 -0.65714286 -0.64285714 -0.62857143 -0.61428571 -0.6 -0.58571429 -0.57142857 -0.55714286 -0.54285714 -0.52857143 -0.51428571 -0.5 -0.48571429 -0.47142857 -0.45714286 -0.44285714 -0.42857143 -0.41428571 -0.4 -0.38571429 -0.37142857 -0.35714286 -0.34285714 -0.32857143 -0.31428571 -0.3 -0.28571429 -0.27142857 -0.25714286 -0.24285714 -0.22857143 -0.21428571 -0.2 -0.18571429 -0.17142857 -0.15714286 -0.14285714 -0.12857143 -0.11428571 -0.1 -0.08571429 -0.07142857 -0.05714286 -0.04285714 -0.02857143 -0.01428571 0 0 0 0 0 0
  line L1 (-6.9437, -1.2061) -> (-6.1524, -1.0687)
  arc A3 (-5.5826, -1.4367) -> (-6.1524, -1.0687) centre (-6.0668, -1.5613) ccw
  arc A4 (-5.5826, -1.4367) -> (-5.3609, -2.1191) centre (0, 0) ccw
  arc A5 (-5.6055, -2.7517) -> (-5.3609, -2.1191) centre (-5.8259, -2.3029) ccw
  line L2 (-5.6055, -2.7517) -> (-6.3265, -3.1056)
  spline S2 degree 5 poles (-6.3265, -3.1056) (-6.3317, -3.1082) (-6.342, -3.1135) (-6.3572, -3.1219) (-6.3768, -3.1341) (-6.4006, -3.1507) (-6.4239, -3.1683) (-6.4468, -3.1864) (-6.4695, -3.2049) (-6.4922, -3.2236) (-6.5147, -3.2426) (-6.537, -3.2619) (-6.5591, -3.2816) (-6.5809, -3.3017) (-6.6024, -3.3224) (-6.6236, -3.3434) (-6.6446, -3.3649) (-6.6654, -3.3866) (-6.686, -3.4086) (-6.7064, -3.4309) (-6.7267, -3.4534) (-6.7468, -3.4763) (-6.7667, -3.4993) (-6.7863, -3.5227) (-6.8058, -3.5464) (-6.8251, -3.5704) (-6.8442, -3.5946) (-6.8631, -3.619) (-6.8819, -3.6437) (-6.9004, -3.6687) (-6.9188, -3.6938) (-6.937, -3.7192) (-6.955, -3.7449) (-6.9729, -3.7707) (-6.9905, -3.7968) (-7.008, -3.8231) (-7.0253, -3.8496) (-7.0425, -3.8764) (-7.0594, -3.9033) (-7.0762, -3.9305) (-7.0928, -3.9578) (-7.1092, -3.9854) (-7.1255, -4.0131) (-7.1415, -4.0411) (-7.1574, -4.0692) (-7.1732, -4.0976) (-7.1887, -4.1261) (-7.2041, -4.1548) (-7.2193, -4.1837) (-7.2343, -4.2127) (-7.2492, -4.242) (-7.2639, -4.2714) (-7.2784, -4.301) (-7.2927, -4.3308) (-7.3068, -4.3608) (-7.3208, -4.3909) (-7.3346, -4.4212) (-7.3482, -4.4516) (-7.3617, -4.4823) (-7.375, -4.5131) (-7.3881, -4.544) (-7.401, -4.5751) (-7.4137, -4.6064) (-7.4263, -4.6378) (-7.4387, -4.6693) (-7.4509, -4.7011) (-7.4629, -4.7329) (-7.4748, -4.765) (-7.4865, -4.7971) (-7.498, -4.8294) (-7.5093, -4.8619) (-7.5182, -4.888) (-7.5249, -4.9076) (-7.5292, -4.9207) (-7.5314, -4.9273) knots 0 0 0 0 0 0 0.01428571 0.02857143 0.04285714 0.05714286 0.07142857 0.08571429 0.1 0.11428571 0.12857143 0.14285714 0.15714286 0.17142857 0.18571429 0.2 0.21428571 0.22857143 0.24285714 0.25714286 0.27142857 0.28571429 0.3 0.31428571 0.32857143 0.34285714 0.35714286 0.37142857 0.38571429 0.4 0.41428571 0.42857143 0.44285714 0.45714286 0.47142857 0.48571429 0.5 0.51428571 0.52857143 0.54285714 0.55714286 0.57142857 0.58571429 0.6 0.61428571 0.62857143 0.64285714 0.65714286 0.67142857 0.68571429 0.7 0.71428571 0.72857143 0.74285714 0.75714286 0.77142857 0.78571429 0.8 0.81428571 0.82857143 0.84285714 0.85714286 0.87142857 0.88571429 0.9 0.91428571 0.92857143 0.94285714 0.95714286 0.97142857 0.98571429 1 1 1 1 1 1
  arc A6 (-7.5314, -4.9273) -> (-7.0134, -5.6402) centre (0, 0) ccw
  spline S3 degree 5 poles (-7.0134, -5.6402) (-7.0065, -5.6401) (-6.9927, -5.64) (-6.972, -5.6398) (-6.9444, -5.6394) (-6.9101, -5.6386) (-6.8758, -5.6377) (-6.8416, -5.6365) (-6.8075, -5.6351) (-6.7734, -5.6335) (-6.7395, -5.6317) (-6.7056, -5.6297) (-6.6719, -5.6274) (-6.6382, -5.625) (-6.6046, -5.6223) (-6.5712, -5.6194) (-6.5378, -5.6163) (-6.5045, -5.613) (-6.4713, -5.6094) (-6.4383, -5.6056) (-6.4053, -5.6017) (-6.3724, -5.5975) (-6.3397, -5.593) (-6.307, -5.5884) (-6.2745, -5.5835) (-6.2421, -5.5784) (-6.2098, -5.5731) (-6.1776, -5.5676) (-6.1456, -5.5619) (-6.1136, -5.5559) (-6.0818, -5.5497) (-6.0501, -5.5433) (-6.0186, -5.5366) (-5.9872, -5.5297) (-5.9559, -5.5226) (-5.9248, -5.5153) (-5.8938, -5.5077) (-5.8629, -5.4999) (-5.8322, -5.4919) (-5.8016, -5.4836) (-5.7712, -5.4751) (-5.7409, -5.4664) (-5.7108, -5.4574) (-5.6809, -5.4482) (-5.6511, -5.4387) (-5.6215, -5.429) (-5.592, -5.4191) (-5.5627, -5.4089) (-5.5336, -5.3984) (-5.5047, -5.3878) (-5.476, -5.3768) (-5.4474, -5.3656) (-5.4191, -5.3541) (-5.391, -5.3423) (-5.3631, -5.3303) (-5.3354, -5.318) (-5.3079, -5.3054) (-5.2806, -5.2926) (-5.2535, -5.2796) (-5.2266, -5.2662) (-5.2, -5.2525) (-5.1737, -5.2385) (-5.1478, -5.224) (-5.1223, -5.2091) (-5.097, -5.1938) (-5.0721, -5.1783) (-5.0473, -5.1625) (-5.0226, -5.1466) (-4.9983, -5.1304) (-4.9744, -5.1137) (-4.9513, -5.0962) (-4.9336, -5.0813) (-4.9209, -5.0695) (-4.9127, -5.0613) (-4.9086, -5.0572) knots -1 -1 -1 -1 -1 -1 -0.98571429 -0.97142857 -0.95714286 -0.94285714 -0.92857143 -0.91428571 -0.9 -0.88571429 -0.87142857 -0.85714286 -0.84285714 -0.82857143 -0.81428571 -0.8 -0.78571429 -0.77142857 -0.75714286 -0.74285714 -0.72857143 -0.71428571 -0.7 -0.68571429 -0.67142857 -0.65714286 -0.64285714 -0.62857143 -0.61428571 -0.6 -0.58571429 -0.57142857 -0.55714286 -0.54285714 -0.52857143 -0.51428571 -0.5 -0.48571429 -0.47142857 -0.45714286 -0.44285714 -0.42857143 -0.41428571 -0.4 -0.38571429 -0.37142857 -0.35714286 -0.34285714 -0.32857143 -0.31428571 -0.3 -0.28571429 -0.27142857 -0.25714286 -0.24285714 -0.22857143 -0.21428571 -0.2 -0.18571429 -0.17142857 -0.15714286 -0.14285714 -0.12857143 -0.11428571 -0.1 -0.08571429 -0.07142857 -0.05714286 -0.04285714 -0.02857143 -0.01428571 0 0 0 0 0 0
  line L3 (-4.9086, -5.0572) -> (-4.3492, -4.4809)
  arc A7 (-3.672, -4.4437) -> (-4.3492, -4.4809) centre (-3.9905, -4.8291) ccw
  arc A8 (-3.672, -4.4437) -> (-3.0915, -4.8654) centre (0, 0) ccw
  arc A9 (-2.9176, -5.521) -> (-3.0915, -4.8654) centre (-3.3596, -5.2874) ccw
  line L4 (-2.9176, -5.521) -> (-3.2928, -6.2312)
  spline S4 degree 5 poles (-3.2928, -6.2312) (-3.2955, -6.2363) (-3.3008, -6.2466) (-3.3081, -6.2623) (-3.3168, -6.2838) (-3.3263, -6.3112) (-3.3348, -6.339) (-3.3426, -6.3672) (-3.3502, -6.3955) (-3.3575, -6.424) (-3.3645, -6.4526) (-3.3713, -6.4813) (-3.3775, -6.5102) (-3.3833, -6.5393) (-3.3886, -6.5686) (-3.3934, -6.5981) (-3.3978, -6.6278) (-3.4018, -6.6576) (-3.4055, -6.6876) (-3.409, -6.7176) (-3.4121, -6.7477) (-3.415, -6.778) (-3.4175, -6.8084) (-3.4196, -6.8389) (-3.4215, -6.8695) (-3.423, -6.9002) (-3.4242, -6.931) (-3.4252, -6.9619) (-3.4258, -6.9929) (-3.4262, -7.024) (-3.4262, -7.0551) (-3.426, -7.0864) (-3.4256, -7.1177) (-3.4248, -7.1491) (-3.4238, -7.1806) (-3.4224, -7.2122) (-3.4208, -7.2438) (-3.419, -7.2755) (-3.4169, -7.3073) (-3.4145, -7.3391) (-3.4118, -7.371) (-3.4089, -7.4029) (-3.4058, -7.4349) (-3.4023, -7.467) (-3.3987, -7.4991) (-3.3947, -7.5313) (-3.3906, -7.5635) (-3.3861, -7.5958) (-3.3814, -7.6281) (-3.3765, -7.6604) (-3.3713, -7.6928) (-3.3659, -7.7253) (-3.3602, -7.7577) (-3.3543, -7.7902) (-3.3482, -7.8228) (-3.3418, -7.8554) (-3.3351, -7.888) (-3.3282, -7.9206) (-3.3211, -7.9533) (-3.3138, -7.986) (-3.3062, -8.0188) (-3.2983, -8.0515) (-3.2903, -8.0843) (-3.282, -8.1171) (-3.2735, -8.1499) (-3.2647, -8.1828) (-3.2557, -8.2156) (-3.2465, -8.2485) (-3.237, -8.2814) (-3.2273, -8.3143) (-3.2174, -8.3472) (-3.2093, -8.3736) (-3.2031, -8.3933) (-3.199, -8.4065) (-3.1969, -8.4131) knots 0 0 0 0 0 0 0.01428571 0.02857143 0.04285714 0.05714286 0.07142857 0.08571429 0.1 0.11428571 0.12857143 0.14285714 0.15714286 0.17142857 0.18571429 0.2 0.21428571 0.22857143 0.24285714 0.25714286 0.27142857 0.28571429 0.3 0.31428571 0.32857143 0.34285714 0.35714286 0.37142857 0.38571429 0.4 0.41428571 0.42857143 0.44285714 0.45714286 0.47142857 0.48571429 0.5 0.51428571 0.52857143 0.54285714 0.55714286 0.57142857 0.58571429 0.6 0.61428571 0.62857143 0.64285714 0.65714286 0.67142857 0.68571429 0.7 0.71428571 0.72857143 0.74285714 0.75714286 0.77142857 0.78571429 0.8 0.81428571 0.82857143 0.84285714 0.85714286 0.87142857 0.88571429 0.9 0.91428571 0.92857143 0.94285714 0.95714286 0.97142857 0.98571429 1 1 1 1 1 1
  arc A10 (-3.1969, -8.4131) -> (-2.3588, -8.6854) centre (0, 0) ccw
  spline S5 degree 5 poles (-2.3588, -8.6854) (-2.3532, -8.6813) (-2.3421, -8.6731) (-2.3255, -8.6607) (-2.3034, -8.6442) (-2.276, -8.6234) (-2.2489, -8.6025) (-2.2219, -8.5814) (-2.1951, -8.5602) (-2.1685, -8.5389) (-2.1421, -8.5175) (-2.1159, -8.496) (-2.0899, -8.4743) (-2.0641, -8.4525) (-2.0386, -8.4306) (-2.0132, -8.4086) (-1.988, -8.3865) (-1.963, -8.3642) (-1.9383, -8.3419) (-1.9137, -8.3194) (-1.8894, -8.2968) (-1.8653, -8.2741) (-1.8414, -8.2512) (-1.8177, -8.2283) (-1.7943, -8.2052) (-1.771, -8.1821) (-1.748, -8.1588) (-1.7252, -8.1354) (-1.7027, -8.1119) (-1.6804, -8.0883) (-1.6583, -8.0646) (-1.6364, -8.0408) (-1.6148, -8.0168) (-1.5934, -7.9928) (-1.5723, -7.9687) (-1.5514, -7.9444) (-1.5308, -7.9201) (-1.5104, -7.8956) (-1.4903, -7.8711) (-1.4704, -7.8464) (-1.4508, -7.8217) (-1.4314, -7.7968) (-1.4124, -7.7719) (-1.3936, -7.7468) (-1.375, -7.7216) (-1.3568, -7.6964) (-1.3388, -7.671) (-1.3211, -7.6456) (-1.3037, -7.62) (-1.2865, -7.5944) (-1.2697, -7.5686) (-1.2532, -7.5428) (-1.2371, -7.5168) (-1.2212, -7.4908) (-1.2058, -7.4646) (-1.1906, -7.4384) (-1.1757, -7.4121) (-1.1611, -7.3857) (-1.1469, -7.3592) (-1.133, -7.3326) (-1.1195, -7.3059) (-1.1065, -7.2791) (-1.0941, -7.2521) (-1.0822, -7.225) (-1.0708, -7.1978) (-1.0597, -7.1706) (-1.0489, -7.1433) (-1.0383, -7.1159) (-1.0281, -7.0885) (-1.0186, -7.061) (-1.0102, -7.0332) (-1.0046, -7.0108) (-1.0013, -6.9937) (-0.9995, -6.9823) (-0.9986, -6.9766) knots -1 -1 -1 -1 -1 -1 -0.98571429 -0.97142857 -0.95714286 -0.94285714 -0.92857143 -0.91428571 -0.9 -0.88571429 -0.87142857 -0.85714286 -0.84285714 -0.82857143 -0.81428571 -0.8 -0.78571429 -0.77142857 -0.75714286 -0.74285714 -0.72857143 -0.71428571 -0.7 -0.68571429 -0.67142857 -0.65714286 -0.64285714 -0.62857143 -0.61428571 -0.6 -0.58571429 -0.57142857 -0.55714286 -0.54285714 -0.52857143 -0.51428571 -0.5 -0.48571429 -0.47142857 -0.45714286 -0.44285714 -0.42857143 -0.41428571 -0.4 -0.38571429 -0.37142857 -0.35714286 -0.34285714 -0.32857143 -0.31428571 -0.3 -0.28571429 -0.27142857 -0.25714286 -0.24285714 -0.22857143 -0.21428571 -0.2 -0.18571429 -0.17142857 -0.15714286 -0.14285714 -0.12857143 -0.11428571 -0.1 -0.08571429 -0.07142857 -0.05714286 -0.04285714 -0.02857143 -0.01428571 0 0 0 0 0 0
  line L5 (-0.9986, -6.9766) -> (-0.8848, -6.1815)
  arc A11 (-0.3588, -5.7533) -> (-0.8848, -6.1815) centre (-0.3899, -6.2524) ccw
  arc A12 (-0.3588, -5.7533) -> (0.3588, -5.7533) centre (0, 0) ccw
  arc A13 (0.8848, -6.1815) -> (0.3588, -5.7533) centre (0.3899, -6.2524) ccw
  line L6 (0.8848, -6.1815) -> (0.9986, -6.9766)
  spline S6 degree 5 poles (0.9986, -6.9766) (0.9995, -6.9823) (1.0013, -6.9937) (1.0046, -7.0108) (1.0102, -7.0332) (1.0186, -7.061) (1.0281, -7.0885) (1.0383, -7.1159) (1.0489, -7.1433) (1.0597, -7.1706) (1.0708, -7.1978) (1.0822, -7.225) (1.0941, -7.2521) (1.1065, -7.2791) (1.1195, -7.3059) (1.133, -7.3326) (1.1469, -7.3592) (1.1611, -7.3857) (1.1757, -7.4121) (1.1906, -7.4384) (1.2058, -7.4646) (1.2212, -7.4908) (1.2371, -7.5168) (1.2532, -7.5428) (1.2697, -7.5686) (1.2865, -7.5944) (1.3037, -7.62) (1.3211, -7.6456) (1.3388, -7.671) (1.3568, -7.6964) (1.375, -7.7216) (1.3936, -7.7468) (1.4124, -7.7719) (1.4314, -7.7968) (1.4508, -7.8217) (1.4704, -7.8464) (1.4903, -7.8711) (1.5104, -7.8956) (1.5308, -7.9201) (1.5514, -7.9444) (1.5723, -7.9687) (1.5934, -7.9928) (1.6148, -8.0168) (1.6364, -8.0408) (1.6583, -8.0646) (1.6804, -8.0883) (1.7027, -8.1119) (1.7252, -8.1354) (1.748, -8.1588) (1.771, -8.1821) (1.7943, -8.2052) (1.8177, -8.2283) (1.8414, -8.2512) (1.8653, -8.2741) (1.8894, -8.2968) (1.9137, -8.3194) (1.9383, -8.3419) (1.963, -8.3642) (1.988, -8.3865) (2.0132, -8.4086) (2.0386, -8.4306) (2.0641, -8.4525) (2.0899, -8.4743) (2.1159, -8.496) (2.1421, -8.5175) (2.1685, -8.5389) (2.1951, -8.5602) (2.2219, -8.5814) (2.2489, -8.6025) (2.276, -8.6234) (2.3034, -8.6442) (2.3255, -8.6607) (2.3421, -8.6731) (2.3532, -8.6813) (2.3588, -8.6854) knots 0 0 0 0 0 0 0.01428571 0.02857143 0.04285714 0.05714286 0.07142857 0.08571429 0.1 0.11428571 0.12857143 0.14285714 0.15714286 0.17142857 0.18571429 0.2 0.21428571 0.22857143 0.24285714 0.25714286 0.27142857 0.28571429 0.3 0.31428571 0.32857143 0.34285714 0.35714286 0.37142857 0.38571429 0.4 0.41428571 0.42857143 0.44285714 0.45714286 0.47142857 0.48571429 0.5 0.51428571 0.52857143 0.54285714 0.55714286 0.57142857 0.58571429 0.6 0.61428571 0.62857143 0.64285714 0.65714286 0.67142857 0.68571429 0.7 0.71428571 0.72857143 0.74285714 0.75714286 0.77142857 0.78571429 0.8 0.81428571 0.82857143 0.84285714 0.85714286 0.87142857 0.88571429 0.9 0.91428571 0.92857143 0.94285714 0.95714286 0.97142857 0.98571429 1 1 1 1 1 1
  arc A14 (2.3588, -8.6854) -> (3.1969, -8.4131) centre (0, 0) ccw